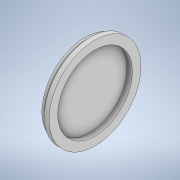
# Autodesk Inventor part: Крышка тих
Saved by Autodesk Inventor 2021 (Build 250183000, 183)
## iProperties
Created: 2023-04-26
Part Number: Крышка тих
Material: Типовые
Document SubType Name: Modeling
Designer: gdevc
Density: 1 g/cm^3
Appearance: По умолчанию
Mass: 44.5921 g
Surface Area: 191.038 cm^2
Volume: 44.5921 cm^3
Author: gdevc
Autodesk Inventor part; units mm, degrees
ref_plane "YZ Plane" through (0, 0, 0) normal (1, 0, 0) x (0, 1, 0)
ref_plane "XZ Plane" through (0, 0, 0) normal (0, 1, 0) x (-1, 0, 0)
ref_plane "XY Plane" through (0, 0, 0) normal (0, 0, 1) x (1, 0, 0)
sketch "Эскиз1" plane through (0, 0, 0) normal (0, 0, 1) x (1, 0, 0)
  line L0 (0, 0) -> (6.2046, 0)
  line L1 (0, 0) -> (0, 45)
  line L2 (0, 45) -> (2.55, 45)
  line L3 (2.55, 45) -> (3.05, 44.5)
  line L4 (3.05, 44.5) -> (5.55, 44.5)
  line L5 (5.55, 44.5) -> (5.55, 48)
  line L6 (5.55, 48) -> (10.55, 48)
  line L7 (10.55, 48) -> (10.55, 39)
  line L8 (10.55, 39) -> (5, 39)
  line L9 (5, 39) -> (5, 0)
  line L10 (0, 0) -> (5, 0)
  dimension "d0" = 45
  dimension "d1" = 0.5
  dimension "d2" = 90
  dimension "d3" = 10.55
  dimension "d4" = 5
  dimension "d5" = 9
  dimension "d6" = 3
  dimension "d7" = 2.5
  dimension "d8" = 5
  constraints: 22 end point, 6 perpendicular, 1 collinear, 1 horizontal, 1 parallel, 1 point on line, 1 vertical
  measures "d0" angle of L2 L3
  measures "d1" distance between parallel lines of L4 L2
  measures "d2" diameter of L2 L0
  measures "d3" distance between parallel lines of L7 L1
  measures "d4" distance between parallel lines of L7 L5
  measures "d5" distance between parallel lines of L6 L8
  measures "d6" distance between parallel lines of L2 L6
  measures "d7" distance of L3.end L4.end
  measures "d8" distance between parallel lines of L1 L9
revolve "Вращение1" add sketch "Эскиз1" angle 360 about axis through (0, 0, 0) along (1, 0, 0)
